Autodesk Inventor part; units mm, degrees
(part 2 of 3)
extrude "Extrusion2" add sketch "Sketch3" against normal blind 0.4 separate body contours L3 L359 L358 L357 L356 L348 L347 L346 L342 L343 L344 L1 L360 L361 L362 L363 L355 L354 L353 L352 L351 L350 | L26 L58 L60 L56 L37 L55 L59 L57 L39 L29 | L67 L70 L63 L171 L170 L162 L163 L72 L164 L161 L71 | L107 L104 L103 L99 L101 L100 L105 L106 L98 | L38 L40 L61 L93 L94 L62 L54 L36 | L73 L78 L168 L82 L166 L167 L165 L83 L74 L81 L80 L79 L77 L76 L75 | L96 L92 A12 A13 L87 | L187 L242 L230 L235 L282 L283 L243 L239 L244 L267 | L270 L271 L272 L274 L276 L277 L278 L275 L273 L268 L269 | L300 L309 L308 L307 L302 L303 L301 L305 L306 | L238 L247 L248 L258 L263 L312 L241 L240 | L249 A39 A42 L262 L264 | L255 L313 L314 L315 L316 L320 L321 L322 L324 L325 L323 L319 L317 L318
sketch "Sketch4" plane through (0, 0, 0.4) normal (0, 0, 1) x (1, 0, 0)
  line L0 (0, 0) -> (63.5, 0)
  line L1 (63.5, 0) -> (63.5, 88.9)
  line L2 (63.5, 88.9) -> (0, 88.9)
  line L3 (0, 88.9) -> (0, 0)
  line L4 (22.2343, 58.9536) -> (21.4951, 58.9536)
  line L5 (22.6153, 59.3346) -> (22.6153, 58.9536)
  line L6 (22.6153, 57.4638) -> (22.6153, 58.9536)
  line L7 (21.4951, 59.3346) -> (22.2343, 59.3346)
  line L8 (21.4951, 52.5322) -> (21.4951, 52.9132)
  line L9 (21.4951, 52.278) -> (21.4951, 58.9536)
  line L10 (21.4951, 52.9132) -> (25.9629, 52.9132)
  line L11 (25.9629, 52.5322) -> (21.4951, 52.5322)
  line L12 (22.6153, 54.7316) -> (22.6153, 57.0828)
  line L13 (22.2343, 58.9536) -> (22.2343, 54.7316)
  circle A0 centre (22.4248, 54.0266) radius 0.3493
  arc A1 (22.2343, 54.7316) -> (22.6153, 54.7316) centre (22.4248, 54.0266) ccw
  line L14 (39.1584, 66.1004) -> (42.0481, 64.4224)
  line L15 (38.6905, 66.1004) -> (39.1584, 66.1004)
  line L16 (38.3095, 62.9084) -> (38.3095, 66.1004)
  line L17 (38.6905, 66.1004) -> (38.6905, 61.5459)
  line L18 (38.3095, 62.9084) -> (37.0962, 62.9084)
  line L19 (37.0962, 62.5274) -> (38.3095, 62.5274)
  line L20 (35.5951, 66.1004) -> (38.3095, 66.1004)
  line L21 (35.2141, 65.0547) -> (35.2141, 66.1004)
  circle A2 centre (38.5, 60.6778) radius 0.508
  circle A3 centre (35.4046, 64.3169) radius 0.3175
  arc A4 (35.2141, 65.0547) -> (35.5951, 65.0547) centre (35.4046, 64.3169) ccw
  line L22 (31.9876, 66.1004) -> (35.2141, 66.1004)
  arc A5 (31.6066, 65.8741) -> (31.9876, 65.8741) centre (31.7971, 65.0383) ccw
  line L23 (35.5951, 66.1004) -> (35.5951, 65.0547)
  line L24 (22.6153, 57.4638) -> (26.9185, 57.4638)
  line L25 (26.9185, 57.0828) -> (22.6153, 57.0828)
  line L26 (26.9185, 57.4638) -> (26.9185, 57.0828)
  circle A6 centre (26.1534, 51.0373) radius 0.4762
  arc A7 (25.9629, 51.8703) -> (26.3439, 51.8703) centre (26.1534, 51.0373) ccw
  line L27 (26.3439, 52.4415) -> (26.3439, 51.8703)
  line L28 (25.9629, 51.8703) -> (25.9629, 52.5322)
  line L29 (26.9185, 55.4481) -> (26.9185, 55.0671)
  line L30 (26.3439, 55.0671) -> (26.3439, 52.8489)
  line L31 (26.9185, 55.0671) -> (26.3439, 55.0671)
  line L32 (25.9629, 52.9132) -> (25.9629, 55.4481)
  line L33 (25.9629, 55.0671) -> (25.9629, 55.4481)
  line L34 (25.9629, 55.4481) -> (26.3439, 55.4481)
  line L35 (25.9629, 55.4481) -> (26.9185, 55.4481)
  line L36 (30.5373, 53.737) -> (30.8468, 54.4929)
  line L37 (29.1789, 54.753) -> (28.0615, 54.753)
  line L38 (29.3943, 53.737) -> (30.5373, 53.737)
  line L39 (26.9185, 54.753) -> (26.9185, 53.737)
  line L40 (29.3943, 53.737) -> (30.8468, 57.9141)
  line L41 (22.2343, 61.6532) -> (25.4283, 64.441)
  line L42 (22.6153, 61.5038) -> (25.4283, 63.959)
  line L43 (25.8093, 61.5568) -> (25.8093, 60.5021)
  line L44 (25.4283, 60.075) -> (25.4283, 60.0896)
  line L45 (25.4283, 60.5021) -> (25.4283, 63.959)
  line L46 (25.8093, 64.9028) -> (25.8093, 61.9378)
  line L47 (25.4283, 64.441) -> (25.4283, 64.9028)
  line L48 (25.4283, 64.9028) -> (22.3363, 64.9028)
  line L49 (21.4951, 59.3346) -> (21.4951, 64.4169)
  line L50 (21.4951, 64.4169) -> (22.3363, 64.9028)
  circle A8 centre (25.6188, 59.7969) radius 0.3493
  line L51 (31.0435, 55.3657) -> (31.9218, 55.3657)
  line L52 (31.4818, 56.4223) -> (31.0435, 55.3657)
  line L53 (31.9218, 55.3657) -> (31.4818, 56.4223)
  line L54 (30.8468, 54.4929) -> (32.1168, 54.4929)
  line L55 (29.1789, 53.737) -> (29.1789, 54.753)
  line L56 (28.0615, 57.9141) -> (28.0615, 54.753)
  line L57 (28.0615, 53.737) -> (26.9185, 53.737)
  line L58 (26.9185, 53.737) -> (26.9185, 57.9141)
  line L59 (26.9185, 53.737) -> (29.1789, 53.737)
  line L60 (26.9185, 57.9141) -> (28.0615, 57.9141)
  line L61 (30.8468, 57.9141) -> (32.1168, 57.9141)
  line L62 (32.4486, 53.737) -> (32.1168, 54.4929)
  line L63 (28.0615, 63.1194) -> (26.9185, 63.1194)
  line L64 (25.8093, 61.9378) -> (26.9185, 61.9378)
  line L65 (26.9185, 61.5568) -> (25.8093, 61.5568)
  line L66 (25.8093, 61.5568) -> (25.8093, 61.6173)
  line L67 (26.9185, 61.9378) -> (26.9185, 61.5568)
  line L68 (22.2343, 59.3346) -> (22.2343, 61.6532)
  line L69 (22.6153, 61.5038) -> (22.6153, 59.3346)
  arc A9 (25.4283, 60.5021) -> (25.8093, 60.5021) centre (25.6188, 59.7969) ccw
  line L70 (26.9185, 63.1194) -> (26.9185, 58.9484)
  line L71 (26.9185, 58.9484) -> (28.0615, 58.9484)
  line L72 (30.9581, 58.9484) -> (29.8151, 58.9484)
  line L73 (32.6087, 58.9484) -> (31.4657, 58.9484)
  line L74 (32.6087, 61.5255) -> (33.8556, 61.5255)
  line L75 (31.4657, 58.9484) -> (33.8556, 58.9484)
  line L76 (33.8556, 58.9484) -> (33.8556, 60.0914)
  line L77 (33.8556, 60.0914) -> (32.6087, 60.0914)
  line L78 (31.4657, 60.0914) -> (31.4657, 58.9484)
  line L79 (32.6087, 60.5095) -> (32.6087, 60.0914)
  line L80 (33.8556, 60.5095) -> (32.6087, 60.5095)
  line L81 (33.8556, 61.5255) -> (33.8556, 60.5095)
  line L82 (31.4657, 60.5095) -> (31.4657, 61.5255)
  line L83 (32.6087, 61.9764) -> (32.6087, 61.5255)
  line L84 (35.0032, 56.9462) -> (35.4388, 56.9462)
  line L85 (35.0032, 54.6929) -> (35.5896, 54.6929)
  line L86 (35.0032, 55.4427) -> (35.5978, 55.4427)
  line L87 (33.911, 53.737) -> (35.876, 53.737)
  line L88 (31.5408, 49.4741) -> (31.5408, 46.3613)
  line L89 (31.9218, 46.3613) -> (31.9218, 48.7095)
  line L90 (31.9218, 46.3613) -> (31.9218, 46.3281)
  line L91 (35.0032, 56.2657) -> (35.0032, 56.9462)
  line L92 (33.911, 57.9141) -> (35.876, 57.9141)
  line L93 (33.5916, 53.737) -> (32.1168, 57.9141)
  line L94 (32.4486, 53.737) -> (33.5916, 53.737)
  line L95 (35.0032, 56.2657) -> (35.4388, 56.2657)
  line L96 (33.911, 53.737) -> (33.911, 57.9141)
  arc A10 (35.4388, 56.2657) -> (35.4388, 56.9462) centre (35.3333, 56.606) ccw
  line L97 (35.0032, 54.6929) -> (35.0032, 55.4427)
  arc A11 (35.5896, 54.6929) -> (35.5978, 55.4427) centre (35.5605, 55.0681) ccw
  arc A12 (36.3387, 56.0044) -> (35.876, 57.9141) centre (35.6477, 56.8479) ccw
  arc A13 (35.876, 53.737) -> (36.3387, 56.0044) centre (35.9369, 54.9055) ccw
  line L98 (37.0962, 62.9084) -> (37.0962, 62.5274)
  line L99 (36.261, 58.9484) -> (35.118, 58.9484)
  line L100 (34.2865, 62.0954) -> (35.118, 62.0954)
  line L101 (35.118, 58.9484) -> (35.118, 62.0954)
  line L102 (35.118, 62.0954) -> (35.2141, 62.0954)
  line L103 (36.261, 62.0954) -> (36.261, 58.9484)
  line L104 (36.261, 62.0954) -> (37.0962, 62.0954)
  line L105 (34.2865, 63.1114) -> (34.2865, 62.0954)
  line L106 (37.0962, 63.1114) -> (34.2865, 63.1114)
  line L107 (37.0962, 62.0954) -> (37.0962, 63.1114)
  line L108 (31.7966, 44.45) -> (43.5019, 51.0525)
  line L109 (42.4624, 51.6596) -> (31.8107, 45.6515)
  line L110 (42.0481, 52.1761) -> (31.9218, 46.3281)
  line L111 (31.9218, 49.1234) -> (37.7054, 52.5185)
  line L112 (31.9218, 48.7095) -> (38.0845, 52.3272)
  line L113 (31.9218, 49.1234) -> (31.9218, 51.0535)
  line L114 (29.0948, 67.2715) -> (29.0948, 67.5351)
  line L115 (29.4758, 67.2715) -> (31.6066, 68.502)
  line L116 (29.0948, 67.5351) -> (31.6066, 68.9857)
  line L117 (31.6066, 65.8741) -> (31.6066, 68.502)
  line L118 (31.6066, 68.9857) -> (31.6066, 70.2564)
  circle A14 centre (29.2853, 63.9396) radius 0.3175
  arc A15 (29.0948, 64.6116) -> (29.4758, 64.6116) centre (29.2853, 63.9396) ccw
  line L119 (29.0948, 64.9028) -> (29.0948, 64.6116)
  line L120 (29.0948, 64.9028) -> (25.8093, 64.9028)
  line L121 (22.9961, 65.2838) -> (29.0948, 65.2838)
  line L122 (29.4758, 64.6116) -> (29.4758, 67.2715)
  line L123 (29.0948, 67.2715) -> (29.0948, 65.2838)
  line L124 (22.9961, 65.2838) -> (31.6066, 70.2564)
  line L125 (31.9876, 66.1004) -> (31.9876, 65.8741)
  line L126 (31.9911, 70.2625) -> (31.9911, 66.4814)
  line L127 (20.9808, 64.9373) -> (31.7409, 71.0066)
  circle A16 centre (31.7971, 65.0383) radius 0.4127
  line L128 (31.75, 72.2052) -> (19.9413, 65.5444)
  line L129 (20.9808, 52.1009) -> (20.9808, 64.9373)
  line L130 (19.9413, 65.5444) -> (19.9413, 51.51)
  circle A17 centre (31.7313, 51.824) radius 0.4127
  line L131 (31.5408, 46.3613) -> (21.4951, 52.278)
  line L132 (19.9413, 51.51) -> (31.7966, 44.45)
  line L133 (31.8107, 45.6515) -> (20.9808, 52.1009)
  line L134 (31.5408, 49.8815) -> (26.3439, 52.8489)
  line L135 (26.3439, 52.4415) -> (31.5408, 49.4741)
  line L136 (31.5408, 51.0535) -> (31.5408, 49.8815)
  arc A18 (31.9218, 51.0535) -> (31.5408, 51.0535) centre (31.7313, 51.824) ccw
  circle A19 centre (41.0606, 62.1232) radius 0.381
  line L137 (40.8701, 59.3346) -> (39.5527, 59.3346)
  line L138 (39.4243, 58.9536) -> (40.8701, 58.9536)
  line L139 (37.7054, 52.5185) -> (37.7054, 53.0908)
  circle A20 centre (37.8959, 53.9267) radius 0.4763
  line L140 (38.7282, 53.737) -> (42.0481, 53.737)
  line L141 (38.0845, 53.0941) -> (38.0845, 52.3272)
  arc A21 (38.7317, 54.1172) -> (37.7054, 53.0908) centre (37.8959, 53.9267) ccw
  arc A22 (38.0845, 53.0941) -> (38.7282, 53.737) centre (37.8959, 53.9267) ccw
  line L142 (42.0481, 53.737) -> (42.0481, 52.1761)
  line L143 (43.5019, 51.0525) -> (43.5019, 65.3384)
  line L144 (42.4624, 64.7418) -> (42.4624, 51.6596)
  line L145 (41.2511, 61.3863) -> (41.2511, 54.1172)
  line L146 (39.4243, 58.9536) -> (38.6183, 59.7969)
  line L147 (39.5527, 59.3346) -> (38.9824, 59.9313)
  arc A23 (41.2511, 61.3863) -> (40.8701, 61.3863) centre (41.0606, 62.1232) ccw
  line L148 (38.3095, 61.5459) -> (38.3095, 62.5274)
  arc A24 (38.9824, 59.9313) -> (38.6905, 61.5459) centre (38.5, 60.6778) ccw
  line L149 (40.8701, 59.3346) -> (40.8701, 61.3863)
  line L150 (42.0481, 64.4224) -> (42.0481, 54.1172)
  line L151 (42.0481, 54.1172) -> (41.2511, 54.1172)
  line L152 (40.8701, 54.1172) -> (40.8701, 58.9536)
  line L153 (40.8701, 54.1172) -> (38.7317, 54.1172)
  arc A25 (38.3095, 61.5459) -> (38.6183, 59.7969) centre (38.5, 60.6778) ccw
  line L154 (43.5019, 65.3384) -> (31.75, 72.2052)
  line L155 (31.7409, 71.0066) -> (42.4624, 64.7418)
  line L156 (38.5023, 66.4814) -> (31.9911, 66.4814)
  line L157 (31.9876, 70.2646) -> (38.5023, 66.4814)
  line L158 (31.9911, 66.4814) -> (31.9911, 70.2625)
  line L159 (31.9911, 70.2625) -> (38.5023, 66.4814)
  line L160 (31.9911, 66.4814) -> (38.5023, 66.4814)
  line L161 (28.0615, 58.9484) -> (28.0615, 61.2883)
  line L162 (29.8151, 63.1194) -> (30.9581, 63.1194)
  line L163 (30.9581, 63.1194) -> (30.9581, 58.9484)
  line L164 (29.8151, 58.9484) -> (28.0615, 61.2883)
  line L165 (33.8556, 61.9764) -> (32.6087, 61.9764)
  line L166 (31.4657, 63.1194) -> (33.8556, 63.1194)
  line L167 (33.8556, 63.1194) -> (33.8556, 61.9764)
  line L168 (31.4657, 58.9484) -> (31.4657, 63.1194)
  line L169 (31.4657, 63.1194) -> (32.6087, 63.1194)
  line L170 (29.8151, 60.7795) -> (29.8151, 63.1194)
  line L171 (28.0615, 63.1194) -> (29.8151, 60.7795)
  line L172 (31.4657, 61.9764) -> (31.4657, 63.1194)
  line L173 (22.6601, 31.2964) -> (22.6651, 29.8066)
  line L174 (22.6665, 29.4256) -> (22.6651, 29.8066)
  line L175 (22.6507, 34.0285) -> (22.6587, 31.6774)
  line L176 (21.5243, 35.8431) -> (25.9921, 35.8584)
  line L177 (25.9908, 36.2394) -> (21.523, 36.2241)
  line L178 (22.2842, 29.8053) -> (21.5449, 29.8027)
  line L179 (21.5462, 29.4217) -> (22.2855, 29.4243)
  circle A26 centre (22.4578, 34.7329) radius 0.3493
  arc A27 (22.6507, 34.0285) -> (22.2697, 34.0272) centre (22.4578, 34.7329) ccw
  line L180 (22.2842, 29.8053) -> (22.2697, 34.0272)
  line L181 (21.523, 36.2241) -> (21.5243, 35.8431)
  line L182 (21.0767, 36.7309) -> (21.12, 24.0813)
  line L183 (19.9676, 23.5047) -> (19.9586, 37.4674)
  line L184 (21.5221, 36.4783) -> (21.5449, 29.8027)
  line L185 (26.9619, 31.6921) -> (22.6587, 31.6774)
  line L186 (22.6601, 31.2964) -> (26.9632, 31.3111)
  line L187 (26.9632, 31.3111) -> (26.9619, 31.6921)
  arc A28 (25.8644, 28.2691) -> (25.4834, 28.2678) centre (25.6715, 28.9736) ccw
  circle A29 centre (25.6715, 28.9736) radius 0.3493
  line L188 (31.8713, 16.6404) -> (19.9676, 23.5047)
  line L189 (21.12, 24.0813) -> (31.8964, 17.907)
  line L190 (23.0676, 23.4777) -> (31.6951, 18.5346)
  line L191 (29.165, 23.8796) -> (29.164, 24.1708)
  line L192 (29.1731, 21.5109) -> (29.1663, 23.4986)
  line L193 (29.1731, 21.5109) -> (29.174, 21.2473)
  line L194 (29.545, 24.1721) -> (29.5541, 21.5122)
  line L195 (29.5541, 21.5122) -> (31.6891, 20.289)
  line L196 (29.174, 21.2473) -> (31.6907, 19.8053)
  line L197 (31.6801, 22.9169) -> (31.6891, 20.289)
  line L198 (31.6907, 19.8053) -> (31.6951, 18.5346)
  line L199 (32.0796, 18.5298) -> (32.0667, 22.3109)
  line L200 (32.0618, 22.6919) -> (32.0611, 22.9182)
  circle A30 centre (31.8677, 23.7534) radius 0.4127
  arc A31 (32.0611, 22.9182) -> (31.6801, 22.9169) centre (31.8677, 23.7534) ccw
  circle A32 centre (41.1212, 26.7001) radius 0.381
  arc A33 (40.9282, 27.4363) -> (41.3092, 27.4376) centre (41.1212, 26.7001) ccw
  line L201 (40.9212, 29.488) -> (40.9282, 27.4363)
  circle A34 centre (38.5556, 28.1368) radius 0.508
  line L202 (40.9212, 29.488) -> (39.6037, 29.4835)
  arc A35 (38.7491, 27.2693) -> (39.0355, 28.8849) centre (38.5556, 28.1368) ccw
  line L203 (39.6037, 29.4835) -> (39.0355, 28.8849)
  line L204 (39.474, 29.8641) -> (40.9199, 29.869)
  line L205 (39.474, 29.8641) -> (38.6709, 29.0181)
  line L206 (42.1166, 24.4043) -> (42.0813, 34.7095)
  line L207 (42.562, 24.1393) -> (42.5183, 36.9086)
  line L208 (43.6866, 37.5937) -> (43.6957, 23.5059)
  line L209 (41.3092, 27.4376) -> (41.2843, 34.7068)
  line L210 (40.9033, 34.7055) -> (40.9199, 29.869)
  line L211 (38.7601, 35.0783) -> (42.08, 35.0897)
  line L212 (40.9033, 34.7055) -> (38.7649, 34.6981)
  line L213 (26.9772, 27.2181) -> (25.868, 27.2143)
  line L214 (25.8693, 26.8333) -> (26.9785, 26.8371)
  line L215 (25.868, 27.2143) -> (25.8644, 28.2691)
  line L216 (25.868, 27.2143) -> (25.8682, 27.1538)
  line L217 (22.6739, 27.2564) -> (22.6665, 29.4256)
  line L218 (22.2855, 29.4243) -> (22.2934, 27.1057)
  line L219 (25.4834, 28.2678) -> (25.4952, 24.8108)
  line L220 (22.6739, 27.2564) -> (25.4952, 24.8108)
  line L221 (21.5462, 29.4217) -> (21.5636, 24.3395)
  line L222 (25.8795, 23.8684) -> (25.8693, 26.8333)
  line L223 (25.4985, 23.8671) -> (22.4066, 23.8565)
  line L224 (21.5636, 24.3395) -> (22.4066, 23.8565)
  line L225 (22.2934, 27.1057) -> (25.4969, 24.3288)
  line L226 (25.9921, 35.8584) -> (26.0007, 33.3235)
  line L227 (26.3804, 33.7058) -> (26.3728, 35.924)
  line L228 (25.9885, 36.9013) -> (25.9908, 36.2394)
  line L229 (26.3714, 36.3314) -> (26.3695, 36.9026)
  line L230 (26.9563, 33.3268) -> (26.955, 33.7078)
  line L231 (26.955, 33.7078) -> (26.3804, 33.7058)
  line L232 (25.9994, 33.7045) -> (26.0007, 33.3235)
  line L233 (26.0007, 33.3235) -> (26.3817, 33.3248)
  line L234 (26.0007, 33.3235) -> (26.9563, 33.3268)
  line L235 (26.954, 34.0219) -> (26.9505, 35.0379)
  line L236 (25.4819, 28.6948) -> (25.482, 28.6802)
  line L237 (25.4969, 24.3288) -> (25.4985, 23.8671)
  line L238 (30.5693, 35.0503) -> (30.8814, 34.2954)
  line L239 (29.2143, 34.0297) -> (28.097, 34.0258)
  line L240 (29.4263, 35.0464) -> (30.5693, 35.0503)
  line L241 (29.4263, 35.0464) -> (30.8931, 30.8743)
  line L242 (26.9505, 35.0379) -> (26.9648, 30.8608)
  line L243 (29.2108, 35.0457) -> (29.2143, 34.0297)
  line L244 (28.1078, 30.8647) -> (28.097, 34.0258)
  circle A36 centre (31.7568, 36.9673) radius 0.4127
  line L245 (31.9366, 40.0825) -> (38.1116, 36.4859)
  line L246 (31.938, 39.6686) -> (37.7332, 36.2932)
  line L247 (30.8814, 34.2954) -> (32.1514, 34.2998)
  line L248 (32.4805, 35.0569) -> (32.1514, 34.2998)
  line L249 (33.9429, 35.0619) -> (35.9079, 35.0686)
  line L250 (31.081, 33.4233) -> (31.9594, 33.4263)
  line L251 (31.523, 32.3682) -> (31.081, 33.4233)
  line L252 (31.9594, 33.4263) -> (31.523, 32.3682)
  line L253 (35.0384, 34.1097) -> (35.6249, 34.1117)
  line L254 (35.041, 33.3599) -> (35.6356, 33.3619)
  circle A37 centre (37.9285, 34.8858) radius 0.4763
  arc A38 (37.7351, 35.7209) -> (38.7649, 34.6981) centre (37.9285, 34.8858) ccw
  arc A39 (36.3784, 32.8027) -> (35.9079, 35.0686) centre (35.9728, 33.9003) ccw
  line L255 (33.9054, 29.8503) -> (33.9093, 28.7073)
  line L256 (31.938, 39.6686) -> (31.9446, 37.7385)
  line L257 (35.0461, 31.8563) -> (35.4817, 31.8578)
  line L258 (32.4805, 35.0569) -> (33.6235, 35.0608)
  line L259 (35.0438, 32.5368) -> (35.4794, 32.5383)
  line L260 (35.0384, 34.1097) -> (35.041, 33.3599)
  arc A40 (35.6356, 33.3619) -> (35.6249, 34.1117) centre (35.597, 33.7363) ccw
  line L261 (35.0438, 32.5368) -> (35.0461, 31.8563)
  arc A41 (35.4817, 31.8578) -> (35.4794, 32.5383) centre (35.375, 32.1977) ccw
  arc A42 (35.9222, 30.8915) -> (36.3784, 32.8027) centre (35.6902, 31.9569) ccw
  line L262 (33.9572, 30.8847) -> (35.9222, 30.8915)
  line L263 (33.6235, 35.0608) -> (32.1631, 30.8786)
  line L264 (33.9429, 35.0619) -> (33.9572, 30.8847)
  line L265 (42.0813, 34.7095) -> (41.2843, 34.7068)
  line L266 (42.08, 35.0897) -> (42.0747, 36.6505)
  line L267 (26.9648, 30.8608) -> (28.1078, 30.8647)
  line L268 (28.1256, 25.6594) -> (26.9826, 25.6555)
  line L269 (26.9785, 26.8371) -> (26.9772, 27.2181)
  line L270 (26.9826, 25.6555) -> (26.9683, 29.8265)
  line L271 (26.9683, 29.8265) -> (28.1113, 29.8304)
  line L272 (28.1113, 29.8304) -> (28.1193, 27.4905)
  line L273 (28.1256, 25.6594) -> (29.8712, 28.0053)
  line L274 (29.8649, 29.8364) -> (28.1193, 27.4905)
  line L275 (29.8712, 28.0053) -> (29.8792, 25.6654)
  line L276 (31.0079, 29.8403) -> (29.8649, 29.8364)
  line L277 (31.0222, 25.6693) -> (31.0079, 29.8403)
  circle A43 centre (29.3522, 24.8434) radius 0.3175
  line L278 (29.8792, 25.6654) -> (31.0222, 25.6693)
  arc A44 (29.545, 24.1721) -> (29.164, 24.1708) centre (29.3522, 24.8434) ccw
  line L279 (38.3728, 25.9055) -> (38.3837, 22.7135)
  line L280 (38.7647, 22.7148) -> (38.7491, 27.2693)
  line L281 (38.3681, 27.268) -> (38.3715, 26.2865)
  circle A45 centre (26.1761, 37.735) radius 0.4762
  arc A46 (26.3695, 36.9026) -> (25.9885, 36.9013) centre (26.1761, 37.735) ccw
  line L282 (28.0935, 35.0418) -> (26.9505, 35.0379)
  line L283 (26.9505, 35.0379) -> (29.2108, 35.0457)
  line L284 (31.5582, 39.3166) -> (31.5476, 42.4293)
  line L285 (31.5596, 38.9092) -> (26.3728, 35.924)
  line L286 (26.3714, 36.3314) -> (31.5582, 39.3166)
  line L287 (31.5476, 42.4293) -> (21.5221, 36.4783)
  line L288 (31.7603, 43.0725) -> (21.0767, 36.7309)
  line L289 (19.9586, 37.4674) -> (31.7966, 44.45)
  line L290 (31.9286, 42.4307) -> (31.9366, 40.0825)
  line L291 (31.9286, 42.4307) -> (31.9285, 42.4639)
  line L292 (31.7966, 44.45) -> (43.6866, 37.5937)
  line L293 (42.5183, 36.9086) -> (31.7603, 43.0725)
  line L294 (42.0747, 36.6505) -> (31.9285, 42.4639)
  line L295 (31.5636, 37.7372) -> (31.5596, 38.9092)
  arc A47 (31.5636, 37.7372) -> (31.9446, 37.7385) centre (31.7568, 36.9673) ccw
  line L296 (38.1142, 35.719) -> (38.1116, 36.4859)
  arc A48 (38.7601, 35.0783) -> (38.1142, 35.719) centre (37.9285, 34.8858) ccw
  line L297 (37.7332, 36.2932) -> (37.7351, 35.7209)
  line L298 (38.3728, 25.9055) -> (37.1595, 25.9014)
  line L299 (37.1582, 26.2824) -> (38.3715, 26.2865)
  line L300 (37.1595, 25.9014) -> (37.1582, 26.2824)
  line L301 (36.3108, 29.8585) -> (35.1678, 29.8546)
  line L302 (34.347, 26.7047) -> (35.1786, 26.7075)
  line L303 (35.1678, 29.8546) -> (35.1786, 26.7075)
  line L304 (35.1786, 26.7075) -> (35.2746, 26.7079)
  line L305 (36.3215, 26.7115) -> (36.3108, 29.8585)
  line L306 (36.3215, 26.7115) -> (37.1567, 26.7143)
  line L307 (34.3505, 25.6887) -> (34.347, 26.7047)
  line L308 (37.1602, 25.6983) -> (34.3505, 25.6887)
  line L309 (37.1567, 26.7143) -> (37.1602, 25.6983)
  arc A49 (38.6709, 29.0181) -> (38.3681, 27.268) centre (38.5556, 28.1368) ccw
  line L310 (29.165, 23.8796) -> (25.8795, 23.8684)
  line L311 (23.0676, 23.4777) -> (29.1663, 23.4986)
  line L312 (30.8931, 30.8743) -> (32.1631, 30.8786)
  line L313 (33.9093, 28.7073) -> (32.6624, 28.703)
  line L314 (32.6638, 28.2849) -> (32.6624, 28.703)
  line L315 (33.9107, 28.2892) -> (32.6638, 28.2849)
  line L316 (33.9142, 27.2732) -> (33.9107, 28.2892)
  line L317 (32.6585, 29.846) -> (31.5155, 29.8421)
  line L318 (31.5155, 29.8421) -> (33.9054, 29.8503)
  line L319 (31.5194, 28.6991) -> (31.5155, 29.8421)
  line L320 (32.6673, 27.2689) -> (33.9142, 27.2732)
  line L321 (32.6688, 26.818) -> (32.6673, 27.2689)
  line L322 (33.9158, 26.8222) -> (32.6688, 26.818)
  line L323 (31.5155, 29.8421) -> (31.5298, 25.6711)
  line L324 (33.9197, 25.6792) -> (33.9158, 26.8222)
  line L325 (31.5298, 25.6711) -> (33.9197, 25.6792)
  line L326 (31.5298, 25.6711) -> (32.6728, 25.675)
  line L327 (31.5258, 26.8141) -> (31.5298, 25.6711)
  line L328 (31.5208, 28.281) -> (31.5243, 27.265)
  line L329 (39.2326, 22.7164) -> (42.1166, 24.4043)
  line L330 (38.7647, 22.7148) -> (39.2326, 22.7164)
  line L331 (35.6693, 22.7042) -> (38.3837, 22.7135)
  line L332 (35.2848, 23.7486) -> (35.2883, 22.7029)
  circle A50 centre (35.4727, 24.4871) radius 0.3175
  arc A51 (35.6658, 23.7499) -> (35.2848, 23.7486) centre (35.4727, 24.4871) ccw
  line L333 (32.0618, 22.6919) -> (35.2883, 22.7029)
  line L334 (35.6693, 22.7042) -> (35.6658, 23.7499)
  line L335 (38.5779, 22.3332) -> (32.0667, 22.3109)
  line L336 (32.0667, 22.3109) -> (38.5779, 22.3332)
  line L337 (31.8964, 17.907) -> (42.562, 24.1393)
  line L338 (43.6957, 23.5059) -> (31.8713, 16.6404)
  line L339 (32.0796, 18.5298) -> (38.5779, 22.3332)
  line L340 (32.0761, 18.5277) -> (38.5779, 22.3332)
  line L341 (32.0667, 22.3109) -> (32.0796, 18.5298)
  line L342 (31.75, 80.4139) -> (44.6823, 72.8573)
  line L343 (44.6823, 72.8573) -> (54.0323, 76.3351)
  line L344 (54.0323, 76.3351) -> (63.5, 70.8029)
  line L345 (31.75, 72.2052) -> (31.75, 88.9) construction
  line L346 (31.75, 80.4139) -> (18.8177, 72.8573)
  line L347 (18.8177, 72.8573) -> (9.4677, 76.3351)
  line L348 (9.4677, 76.3351) -> (0, 70.8029)
  line L349 (29.1432, 44.45) -> (63.5, 44.45) construction
  line L350 (9.4677, 12.5649) -> (0, 18.0971)
  line L351 (18.8177, 16.0427) -> (9.4677, 12.5649)
  line L352 (31.75, 8.4861) -> (18.8177, 16.0427)
  line L353 (31.75, 8.4861) -> (44.6823, 16.0427)
  line L354 (44.6823, 16.0427) -> (54.0323, 12.5649)
  line L355 (54.0323, 12.5649) -> (63.5, 18.0971)
  line L356 (0, 51.1737) -> (17.8526, 51.1737)
  line L357 (17.8526, 51.1737) -> (29.1432, 44.45)
  line L358 (17.8526, 37.7263) -> (29.1432, 44.45)
  line L359 (0, 37.7263) -> (17.8526, 37.7263)
  line L360 (63.5, 51.1737) -> (45.6474, 51.1737)
  line L361 (45.6474, 51.1737) -> (34.3568, 44.45)
  line L362 (45.6474, 37.7263) -> (34.3568, 44.45)
  line L363 (63.5, 37.7263) -> (45.6474, 37.7263)
  point P0 (0, 0)
  point P1 (31.7785, 58.3278)
  point P2 (31.8262, 30.4638)
  point P3 (-41.3099, 18.32)
  point P4 (-51.7367, 24.4909)
  point P5 (-46.8879, 27.4068)
  point P6 (-46.3133, 27.4068)
  point P7 (-46.3133, 29.0414)
  point P8 (-41.2407, 42.2212)
  point P9 (-46.3133, 29.4224)
  point P10 (-45.1703, 25.6956)
  point P11 (-46.3133, 26.7116)
  point P12 (-46.3133, 27.0258)
  point P13 (-36.1356, 34.4861)
  point P14 (-36.1356, 34.8671)
  point P15 (-46.3133, 33.8965)
  point P16 (-46.3133, 33.5155)
  point P17 (-40.6231, 30.9071)
  point P18 (-41.7661, 32.0501)
  point P19 (-41.7661, 32.4682)
  point P20 (-41.3032, 14.3893)
  point P21 (-51.7088, 8.1828)
  point P22 (-46.2698, 3.6508)
  point P23 (-46.2754, 5.2854)
  point P24 (-46.85, 5.2835)
  point P25 (-46.2545, -0.8232)
  point P26 (-46.2532, -1.2042)
  point P27 (-36.0723, -2.1399)
  point P28 (-36.0736, -1.7589)
  point P29 (-46.2767, 5.6664)
  point P30 (-46.2778, 5.9806)
  point P31 (-45.1383, 7.0005)
  point P32 (-46.2685, 3.2698)
  point P33 (-41.7124, 0.6578)
  point P34 (-40.5733, 1.8047)
  point P35 (-9.7318, -9.9442)
  point P36 (-73.2318, -9.9442)
  point P37 (-73.2318, 42.7616)
  dimension "d21" = 63.5
  dimension "d22" = 88.9
  constraints: 728 end point, 89 parallel, 64 point on circle, 50 centre point, 37 horizontal, 22 point on line, 21 perpendicular, 20 coincident, 17 symmetric about line, 5 vertical, 4 collinear, 2 midpoint, 11 other
  measures "d21" distance of L2.end L1.end
  measures "d22" distance of L1.end L0.end
extrude "Extrusion3" add sketch "Sketch4" against normal blind 0.4 separate body contours L3 L356 L357 L358 L359 | L363 L362 L361 L360 L1
sketch "Sketch5" plane through (0, 0, 0) normal (0, 0, -1) x (-1, 0, 0)
  line L0 (-29.8712, 28.0053) -> (-28.1256, 25.6594) projected
  line L1 (-28.1256, 25.6594) -> (-26.9826, 25.6555) projected
  line L2 (-26.9826, 25.6555) -> (-26.9683, 29.8265) projected
  line L3 (-26.9683, 29.8265) -> (-28.1113, 29.8304) projected
  line L4 (-28.1113, 29.8304) -> (-28.1193, 27.4905) projected
  line L5 (-28.1193, 27.4905) -> (-29.8649, 29.8364) projected
  line L6 (-29.8649, 29.8364) -> (-31.0079, 29.8403) projected
  line L7 (-31.0079, 29.8403) -> (-31.0222, 25.6693) projected
  line L8 (-31.0222, 25.6693) -> (-29.8792, 25.6654) projected
  line L9 (-29.8792, 25.6654) -> (-29.8712, 28.0053) projected
  line L10 (-28.097, 34.0258) -> (-28.1078, 30.8647) projected
  line L11 (-28.1078, 30.8647) -> (-26.9648, 30.8608) projected
  line L12 (-26.9648, 30.8608) -> (-26.9505, 35.0379) projected
  line L13 (-26.9505, 35.0379) -> (-29.2108, 35.0457) projected
  line L14 (-29.2108, 35.0457) -> (-29.2143, 34.0297) projected
  line L15 (-29.2143, 34.0297) -> (-28.097, 34.0258) projected
  line L16 (-32.1631, 30.8786) -> (-30.8931, 30.8743) projected
  line L17 (-30.8931, 30.8743) -> (-29.4263, 35.0464) projected
  line L18 (-29.4263, 35.0464) -> (-30.5693, 35.0503) projected
  line L19 (-30.5693, 35.0503) -> (-30.8814, 34.2954) projected
  line L20 (-30.8814, 34.2954) -> (-32.1514, 34.2998) projected
  line L21 (-32.1514, 34.2998) -> (-32.4805, 35.0569) projected
  line L22 (-32.4805, 35.0569) -> (-33.6235, 35.0608) projected
  line L23 (-33.6235, 35.0608) -> (-32.1631, 30.8786) projected
  line L24 (-31.9594, 33.4263) -> (-31.081, 33.4233) projected
  line L25 (-31.081, 33.4233) -> (-31.523, 32.3682) projected
  line L26 (-31.523, 32.3682) -> (-31.9594, 33.4263) projected
  arc A0 (-36.3784, 32.8027) -> (-35.9222, 30.8915) centre (-35.6902, 31.9569) ccw projected
  line L27 (-35.9222, 30.8915) -> (-33.9572, 30.8847) projected
  line L28 (-33.9572, 30.8847) -> (-33.9429, 35.0619) projected
  line L29 (-33.9429, 35.0619) -> (-35.9079, 35.0686) projected
  arc A1 (-35.9079, 35.0686) -> (-36.3784, 32.8027) centre (-35.9728, 33.9003) ccw projected
  line L30 (-35.4794, 32.5383) -> (-35.0438, 32.5368) projected
  line L31 (-35.0438, 32.5368) -> (-35.0461, 31.8563) projected
  line L32 (-35.0461, 31.8563) -> (-35.4817, 31.8578) projected
  arc A2 (-35.4794, 32.5383) -> (-35.4817, 31.8578) centre (-35.375, 32.1977) ccw projected
  line L33 (-35.0384, 34.1097) -> (-35.041, 33.3599) projected
  line L34 (-35.041, 33.3599) -> (-35.6356, 33.3619) projected
  arc A3 (-35.6249, 34.1117) -> (-35.6356, 33.3619) centre (-35.597, 33.7363) ccw projected
  line L35 (-35.6249, 34.1117) -> (-35.0384, 34.1097) projected
  line L36 (-31.5155, 29.8421) -> (-33.9054, 29.8503) projected
  line L37 (-33.9054, 29.8503) -> (-33.9093, 28.7073) projected
  line L38 (-33.9093, 28.7073) -> (-32.6624, 28.703) projected
  line L39 (-32.6624, 28.703) -> (-32.6638, 28.2849) projected
  line L40 (-32.6638, 28.2849) -> (-33.9107, 28.2892) projected
  line L41 (-33.9107, 28.2892) -> (-33.9142, 27.2732) projected
  line L42 (-33.9142, 27.2732) -> (-32.6673, 27.2689) projected
  line L43 (-32.6673, 27.2689) -> (-32.6688, 26.818) projected
  line L44 (-32.6688, 26.818) -> (-33.9158, 26.8222) projected
  line L45 (-33.9158, 26.8222) -> (-33.9197, 25.6792) projected
  line L46 (-33.9197, 25.6792) -> (-31.5298, 25.6711) projected
  line L47 (-31.5298, 25.6711) -> (-31.5155, 29.8421) projected
  line L48 (-36.3108, 29.8585) -> (-36.3215, 26.7115) projected
  line L49 (-36.3215, 26.7115) -> (-37.1567, 26.7143) projected
  line L50 (-37.1567, 26.7143) -> (-37.1602, 25.6983) projected
  line L51 (-37.1602, 25.6983) -> (-34.3505, 25.6887) projected
  line L52 (-34.3505, 25.6887) -> (-34.347, 26.7047) projected
  line L53 (-34.347, 26.7047) -> (-35.1786, 26.7075) projected
  line L54 (-35.1786, 26.7075) -> (-35.1678, 29.8546) projected
  line L55 (-35.1678, 29.8546) -> (-36.3108, 29.8585) projected
  line L56 (-26.9185, 58.9484) -> (-26.9185, 63.1194) projected
  line L57 (-26.9185, 63.1194) -> (-28.0615, 63.1194) projected
  line L58 (-28.0615, 63.1194) -> (-29.8151, 60.7795) projected
  line L59 (-29.8151, 60.7795) -> (-29.8151, 63.1194) projected
  line L60 (-29.8151, 63.1194) -> (-30.9581, 63.1194) projected
  line L61 (-30.9581, 63.1194) -> (-30.9581, 58.9484) projected
  line L62 (-30.9581, 58.9484) -> (-29.8151, 58.9484) projected
  line L63 (-29.8151, 58.9484) -> (-28.0615, 61.2883) projected
  line L64 (-28.0615, 61.2883) -> (-28.0615, 58.9484) projected
  line L65 (-28.0615, 58.9484) -> (-26.9185, 58.9484) projected
  line L66 (-32.6087, 60.0914) -> (-33.8556, 60.0914) projected
  line L67 (-33.8556, 60.0914) -> (-33.8556, 58.9484) projected
  line L68 (-33.8556, 58.9484) -> (-31.4657, 58.9484) projected
  line L69 (-31.4657, 58.9484) -> (-31.4657, 63.1194) projected
  line L70 (-31.4657, 63.1194) -> (-33.8556, 63.1194) projected
  line L71 (-33.8556, 63.1194) -> (-33.8556, 61.9764) projected
  line L72 (-33.8556, 61.9764) -> (-32.6087, 61.9764) projected
  line L73 (-32.6087, 61.9764) -> (-32.6087, 61.5255) projected
  line L74 (-32.6087, 61.5255) -> (-33.8556, 61.5255) projected
  line L75 (-33.8556, 61.5255) -> (-33.8556, 60.5095) projected
  line L76 (-33.8556, 60.5095) -> (-32.6087, 60.5095) projected
  line L77 (-32.6087, 60.5095) -> (-32.6087, 60.0914) projected
  line L78 (-37.0962, 63.1114) -> (-37.0962, 62.0954) projected
  line L79 (-37.0962, 62.0954) -> (-36.261, 62.0954) projected
  line L80 (-36.261, 62.0954) -> (-36.261, 58.9484) projected
  line L81 (-36.261, 58.9484) -> (-35.118, 58.9484) projected
  line L82 (-35.118, 58.9484) -> (-35.118, 62.0954) projected
  line L83 (-35.118, 62.0954) -> (-34.2865, 62.0954) projected
  line L84 (-34.2865, 62.0954) -> (-34.2865, 63.1114) projected
  line L85 (-34.2865, 63.1114) -> (-37.0962, 63.1114) projected
  line L86 (-26.9185, 53.737) -> (-26.9185, 57.9141) projected
  line L87 (-26.9185, 57.9141) -> (-28.0615, 57.9141) projected
  line L88 (-28.0615, 57.9141) -> (-28.0615, 54.753) projected
  line L89 (-28.0615, 54.753) -> (-29.1789, 54.753) projected
  line L90 (-29.1789, 54.753) -> (-29.1789, 53.737) projected
  line L91 (-29.1789, 53.737) -> (-26.9185, 53.737) projected
  line L92 (-30.8468, 54.4929) -> (-30.5373, 53.737) projected
  line L93 (-30.5373, 53.737) -> (-29.3943, 53.737) projected
  line L94 (-29.3943, 53.737) -> (-30.8468, 57.9141) projected
  line L95 (-30.8468, 57.9141) -> (-32.1168, 57.9141) projected
  line L96 (-32.1168, 57.9141) -> (-33.5916, 53.737) projected
  line L97 (-33.5916, 53.737) -> (-32.4486, 53.737) projected
  line L98 (-32.4486, 53.737) -> (-32.1168, 54.4929) projected
  line L99 (-32.1168, 54.4929) -> (-30.8468, 54.4929) projected
  line L100 (-31.4818, 56.4223) -> (-31.0435, 55.3657) projected
  line L101 (-31.0435, 55.3657) -> (-31.9218, 55.3657) projected
  line L102 (-31.9218, 55.3657) -> (-31.4818, 56.4223) projected
  line L103 (-35.876, 53.737) -> (-33.911, 53.737) projected
  line L104 (-33.911, 53.737) -> (-33.911, 57.9141) projected
  line L105 (-33.911, 57.9141) -> (-35.876, 57.9141) projected
  arc A4 (-35.876, 57.9141) -> (-36.3387, 56.0044) centre (-35.6477, 56.8479) ccw projected
  arc A5 (-36.3387, 56.0044) -> (-35.876, 53.737) centre (-35.9369, 54.9055) ccw projected
  line L106 (-35.5978, 55.4427) -> (-35.0032, 55.4427) projected
  line L107 (-35.0032, 55.4427) -> (-35.0032, 54.6929) projected
  line L108 (-35.0032, 54.6929) -> (-35.5896, 54.6929) projected
  arc A6 (-35.5978, 55.4427) -> (-35.5896, 54.6929) centre (-35.5605, 55.0681) ccw projected
  line L109 (-35.0032, 56.9462) -> (-35.0032, 56.2657) projected
  line L110 (-35.0032, 56.2657) -> (-35.4388, 56.2657) projected
  arc A7 (-35.4388, 56.9462) -> (-35.4388, 56.2657) centre (-35.3333, 56.606) ccw projected
  line L111 (-35.4388, 56.9462) -> (-35.0032, 56.9462) projected
  point P0 (0, 0)
extrude "Extrusion4" add sketch "Sketch5" along normal blind 0.4 bodies 2
sketch "Sketch6" plane through (0, 0, 0.4) normal (0, 0, 1) x (1, 0, 0)
  line L0 (0, 0) -> (63.5, 0)
  line L1 (63.5, 0) -> (63.5, 88.9)
  line L2 (63.5, 88.9) -> (0, 88.9)
  line L3 (0, 88.9) -> (0, 0)
  line L4 (22.2343, 58.9536) -> (21.4951, 58.9536)
  line L5 (22.6153, 59.3346) -> (22.6153, 58.9536)
  line L6 (22.6153, 57.4638) -> (22.6153, 58.9536)
  line L7 (21.4951, 59.3346) -> (22.2343, 59.3346)
  line L8 (21.4951, 52.5322) -> (21.4951, 52.9132)
  line L9 (21.4951, 52.278) -> (21.4951, 58.9536)
  line L10 (21.4951, 52.9132) -> (25.9629, 52.9132)
  line L11 (25.9629, 52.5322) -> (21.4951, 52.5322)
  line L12 (22.6153, 54.7316) -> (22.6153, 57.0828)
  line L13 (22.2343, 58.9536) -> (22.2343, 54.7316)
  circle A0 centre (22.4248, 54.0266) radius 0.3493
  arc A1 (22.2343, 54.7316) -> (22.6153, 54.7316) centre (22.4248, 54.0266) ccw
  line L14 (39.1584, 66.1004) -> (42.0481, 64.4224)
  line L15 (38.6905, 66.1004) -> (39.1584, 66.1004)
  line L16 (38.3095, 62.9084) -> (38.3095, 66.1004)
  line L17 (38.6905, 66.1004) -> (38.6905, 61.5459)
  line L18 (38.3095, 62.9084) -> (37.0962, 62.9084)
  line L19 (37.0962, 62.5274) -> (38.3095, 62.5274)
  line L20 (35.5951, 66.1004) -> (38.3095, 66.1004)
  line L21 (35.2141, 65.0547) -> (35.2141, 66.1004)
  circle A2 centre (38.5, 60.6778) radius 0.508
  circle A3 centre (35.4046, 64.3169) radius 0.3175
  arc A4 (35.2141, 65.0547) -> (35.5951, 65.0547) centre (35.4046, 64.3169) ccw
  line L22 (31.9876, 66.1004) -> (35.2141, 66.1004)
  arc A5 (31.6066, 65.8741) -> (31.9876, 65.8741) centre (31.7971, 65.0383) ccw
  line L23 (35.5951, 66.1004) -> (35.5951, 65.0547)
  line L24 (22.6153, 57.4638) -> (26.9185, 57.4638)
  line L25 (26.9185, 57.0828) -> (22.6153, 57.0828)
  line L26 (26.9185, 57.4638) -> (26.9185, 57.0828)
  circle A6 centre (26.1534, 51.0373) radius 0.4762
  arc A7 (25.9629, 51.8703) -> (26.3439, 51.8703) centre (26.1534, 51.0373) ccw
  line L27 (26.3439, 52.4415) -> (26.3439, 51.8703)
  line L28 (25.9629, 51.8703) -> (25.9629, 52.5322)
  line L29 (26.9185, 55.4481) -> (26.9185, 55.0671)
  line L30 (26.3439, 55.0671) -> (26.3439, 52.8489)
  line L31 (26.9185, 55.0671) -> (26.3439, 55.0671)
  line L32 (25.9629, 52.9132) -> (25.9629, 55.4481)
  line L33 (25.9629, 55.0671) -> (25.9629, 55.4481)
  line L34 (25.9629, 55.4481) -> (26.3439, 55.4481)
  line L35 (25.9629, 55.4481) -> (26.9185, 55.4481)
  line L36 (30.5373, 53.737) -> (30.8468, 54.4929)
  line L37 (29.1789, 54.753) -> (28.0615, 54.753)
  line L38 (29.3943, 53.737) -> (30.5373, 53.737)
  line L39 (26.9185, 54.753) -> (26.9185, 53.737)
  line L40 (29.3943, 53.737) -> (30.8468, 57.9141)
  line L41 (22.2343, 61.6532) -> (25.4283, 64.441)
  line L42 (22.6153, 61.5038) -> (25.4283, 63.959)
  line L43 (25.8093, 61.5568) -> (25.8093, 60.5021)
  line L44 (25.4283, 60.075) -> (25.4283, 60.0896)
  line L45 (25.4283, 60.5021) -> (25.4283, 63.959)
  line L46 (25.8093, 64.9028) -> (25.8093, 61.9378)
  line L47 (25.4283, 64.441) -> (25.4283, 64.9028)
  line L48 (25.4283, 64.9028) -> (22.3363, 64.9028)
  line L49 (21.4951, 59.3346) -> (21.4951, 64.4169)
  line L50 (21.4951, 64.4169) -> (22.3363, 64.9028)
  circle A8 centre (25.6188, 59.7969) radius 0.3493
  line L51 (31.0435, 55.3657) -> (31.9218, 55.3657)
  line L52 (31.4818, 56.4223) -> (31.0435, 55.3657)
  line L53 (31.9218, 55.3657) -> (31.4818, 56.4223)
  line L54 (30.8468, 54.4929) -> (32.1168, 54.4929)
  line L55 (29.1789, 53.737) -> (29.1789, 54.753)
  line L56 (28.0615, 57.9141) -> (28.0615, 54.753)
  line L57 (28.0615, 53.737) -> (26.9185, 53.737)
  line L58 (26.9185, 53.737) -> (26.9185, 57.9141)
  line L59 (26.9185, 53.737) -> (29.1789, 53.737)
  line L60 (26.9185, 57.9141) -> (28.0615, 57.9141)
  line L61 (30.8468, 57.9141) -> (32.1168, 57.9141)
  line L62 (32.4486, 53.737) -> (32.1168, 54.4929)
  line L63 (28.0615, 63.1194) -> (26.9185, 63.1194)
  line L64 (25.8093, 61.9378) -> (26.9185, 61.9378)
  line L65 (26.9185, 61.5568) -> (25.8093, 61.5568)
  line L66 (25.8093, 61.5568) -> (25.8093, 61.6173)
  line L67 (26.9185, 61.9378) -> (26.9185, 61.5568)
  line L68 (22.2343, 59.3346) -> (22.2343, 61.6532)
  line L69 (22.6153, 61.5038) -> (22.6153, 59.3346)
  arc A9 (25.4283, 60.5021) -> (25.8093, 60.5021) centre (25.6188, 59.7969) ccw
  line L70 (26.9185, 63.1194) -> (26.9185, 58.9484)
  line L71 (26.9185, 58.9484) -> (28.0615, 58.9484)
  line L72 (30.9581, 58.9484) -> (29.8151, 58.9484)
  line L73 (32.6087, 58.9484) -> (31.4657, 58.9484)
  line L74 (32.6087, 61.5255) -> (33.8556, 61.5255)
  line L75 (31.4657, 58.9484) -> (33.8556, 58.9484)
  line L76 (33.8556, 58.9484) -> (33.8556, 60.0914)
  line L77 (33.8556, 60.0914) -> (32.6087, 60.0914)
  line L78 (31.4657, 60.0914) -> (31.4657, 58.9484)
  line L79 (32.6087, 60.5095) -> (32.6087, 60.0914)
  line L80 (33.8556, 60.5095) -> (32.6087, 60.5095)
  line L81 (33.8556, 61.5255) -> (33.8556, 60.5095)
  line L82 (31.4657, 60.5095) -> (31.4657, 61.5255)
  line L83 (32.6087, 61.9764) -> (32.6087, 61.5255)
  line L84 (35.0032, 56.9462) -> (35.4388, 56.9462)
  line L85 (35.0032, 54.6929) -> (35.5896, 54.6929)
  line L86 (35.0032, 55.4427) -> (35.5978, 55.4427)
  line L87 (33.911, 53.737) -> (35.876, 53.737)
  line L88 (31.5408, 49.4741) -> (31.5408, 46.3613)
  line L89 (31.9218, 46.3613) -> (31.9218, 48.7095)
  line L90 (31.9218, 46.3613) -> (31.9218, 46.3281)
  line L91 (35.0032, 56.2657) -> (35.0032, 56.9462)
  line L92 (33.911, 57.9141) -> (35.876, 57.9141)
  line L93 (33.5916, 53.737) -> (32.1168, 57.9141)
  line L94 (32.4486, 53.737) -> (33.5916, 53.737)
  line L95 (35.0032, 56.2657) -> (35.4388, 56.2657)
  line L96 (33.911, 53.737) -> (33.911, 57.9141)
  arc A10 (35.4388, 56.2657) -> (35.4388, 56.9462) centre (35.3333, 56.606) ccw
  line L97 (35.0032, 54.6929) -> (35.0032, 55.4427)
  arc A11 (35.5896, 54.6929) -> (35.5978, 55.4427) centre (35.5605, 55.0681) ccw
  arc A12 (36.3387, 56.0044) -> (35.876, 57.9141) centre (35.6477, 56.8479) ccw
  arc A13 (35.876, 53.737) -> (36.3387, 56.0044) centre (35.9369, 54.9055) ccw
  line L98 (37.0962, 62.9084) -> (37.0962, 62.5274)
  line L99 (36.261, 58.9484) -> (35.118, 58.9484)
  line L100 (34.2865, 62.0954) -> (35.118, 62.0954)
  line L101 (35.118, 58.9484) -> (35.118, 62.0954)
  line L102 (35.118, 62.0954) -> (35.2141, 62.0954)
  line L103 (36.261, 62.0954) -> (36.261, 58.9484)
  line L104 (36.261, 62.0954) -> (37.0962, 62.0954)
  line L105 (34.2865, 63.1114) -> (34.2865, 62.0954)
  line L106 (37.0962, 63.1114) -> (34.2865, 63.1114)
  line L107 (37.0962, 62.0954) -> (37.0962, 63.1114)
  line L108 (31.7966, 44.45) -> (43.5019, 51.0525)
  line L109 (42.4624, 51.6596) -> (31.8107, 45.6515)
  line L110 (42.0481, 52.1761) -> (31.9218, 46.3281)
  line L111 (31.9218, 49.1234) -> (37.7054, 52.5185)
  line L112 (31.9218, 48.7095) -> (38.0845, 52.3272)
  line L113 (31.9218, 49.1234) -> (31.9218, 51.0535)
  line L114 (29.0948, 67.2715) -> (29.0948, 67.5351)
  line L115 (29.4758, 67.2715) -> (31.6066, 68.502)
  line L116 (29.0948, 67.5351) -> (31.6066, 68.9857)
  line L117 (31.6066, 65.8741) -> (31.6066, 68.502)
  line L118 (31.6066, 68.9857) -> (31.6066, 70.2564)
  circle A14 centre (29.2853, 63.9396) radius 0.3175
  arc A15 (29.0948, 64.6116) -> (29.4758, 64.6116) centre (29.2853, 63.9396) ccw
  line L119 (29.0948, 64.9028) -> (29.0948, 64.6116)
  line L120 (29.0948, 64.9028) -> (25.8093, 64.9028)
  line L121 (22.9961, 65.2838) -> (29.0948, 65.2838)
  line L122 (29.4758, 64.6116) -> (29.4758, 67.2715)
  line L123 (29.0948, 67.2715) -> (29.0948, 65.2838)
  line L124 (22.9961, 65.2838) -> (31.6066, 70.2564)
  line L125 (31.9876, 66.1004) -> (31.9876, 65.8741)
  line L126 (31.9911, 70.2625) -> (31.9911, 66.4814)
  line L127 (20.9808, 64.9373) -> (31.7409, 71.0066)
  circle A16 centre (31.7971, 65.0383) radius 0.4127
  line L128 (31.75, 72.2052) -> (19.9413, 65.5444)
  line L129 (20.9808, 52.1009) -> (20.9808, 64.9373)
  line L130 (19.9413, 65.5444) -> (19.9413, 51.51)
  circle A17 centre (31.7313, 51.824) radius 0.4127
  line L131 (31.5408, 46.3613) -> (21.4951, 52.278)
  line L132 (19.9413, 51.51) -> (31.7966, 44.45)
  line L133 (31.8107, 45.6515) -> (20.9808, 52.1009)
  line L134 (31.5408, 49.8815) -> (26.3439, 52.8489)
  line L135 (26.3439, 52.4415) -> (31.5408, 49.4741)
  line L136 (31.5408, 51.0535) -> (31.5408, 49.8815)
  arc A18 (31.9218, 51.0535) -> (31.5408, 51.0535) centre (31.7313, 51.824) ccw
  circle A19 centre (41.0606, 62.1232) radius 0.381
  line L137 (40.8701, 59.3346) -> (39.5527, 59.3346)
  line L138 (39.4243, 58.9536) -> (40.8701, 58.9536)
  line L139 (37.7054, 52.5185) -> (37.7054, 53.0908)
  circle A20 centre (37.8959, 53.9267) radius 0.4763
  line L140 (38.7282, 53.737) -> (42.0481, 53.737)
  line L141 (38.0845, 53.0941) -> (38.0845, 52.3272)
  arc A21 (38.7317, 54.1172) -> (37.7054, 53.0908) centre (37.8959, 53.9267) ccw
  arc A22 (38.0845, 53.0941) -> (38.7282, 53.737) centre (37.8959, 53.9267) ccw
  line L142 (42.0481, 53.737) -> (42.0481, 52.1761)
  line L143 (43.5019, 51.0525) -> (43.5019, 65.3384)
  line L144 (42.4624, 64.7418) -> (42.4624, 51.6596)
  line L145 (41.2511, 61.3863) -> (41.2511, 54.1172)
  line L146 (39.4243, 58.9536) -> (38.6183, 59.7969)
  line L147 (39.5527, 59.3346) -> (38.9824, 59.9313)
  arc A23 (41.2511, 61.3863) -> (40.8701, 61.3863) centre (41.0606, 62.1232) ccw
  line L148 (38.3095, 61.5459) -> (38.3095, 62.5274)
  arc A24 (38.9824, 59.9313) -> (38.6905, 61.5459) centre (38.5, 60.6778) ccw
  line L149 (40.8701, 59.3346) -> (40.8701, 61.3863)
  line L150 (42.0481, 64.4224) -> (42.0481, 54.1172)
  line L151 (42.0481, 54.1172) -> (41.2511, 54.1172)
  line L152 (40.8701, 54.1172) -> (40.8701, 58.9536)
  line L153 (40.8701, 54.1172) -> (38.7317, 54.1172)
  arc A25 (38.3095, 61.5459) -> (38.6183, 59.7969) centre (38.5, 60.6778) ccw
  line L154 (43.5019, 65.3384) -> (31.75, 72.2052)
  line L155 (31.7409, 71.0066) -> (42.4624, 64.7418)
  line L156 (38.5023, 66.4814) -> (31.9911, 66.4814)
  line L157 (31.9876, 70.2646) -> (38.5023, 66.4814)
  line L158 (31.9911, 66.4814) -> (31.9911, 70.2625)
  line L159 (31.9911, 70.2625) -> (38.5023, 66.4814)
  line L160 (31.9911, 66.4814) -> (38.5023, 66.4814)
  line L161 (28.0615, 58.9484) -> (28.0615, 61.2883)
  line L162 (29.8151, 63.1194) -> (30.9581, 63.1194)
  line L163 (30.9581, 63.1194) -> (30.9581, 58.9484)
  line L164 (29.8151, 58.9484) -> (28.0615, 61.2883)
  line L165 (33.8556, 61.9764) -> (32.6087, 61.9764)
  line L166 (31.4657, 63.1194) -> (33.8556, 63.1194)
  line L167 (33.8556, 63.1194) -> (33.8556, 61.9764)
  line L168 (31.4657, 58.9484) -> (31.4657, 63.1194)
  line L169 (31.4657, 63.1194) -> (32.6087, 63.1194)
  line L170 (29.8151, 60.7795) -> (29.8151, 63.1194)
  line L171 (28.0615, 63.1194) -> (29.8151, 60.7795)
  line L172 (31.4657, 61.9764) -> (31.4657, 63.1194)
  line L173 (22.6601, 31.2964) -> (22.6651, 29.8066)
  line L174 (22.6665, 29.4256) -> (22.6651, 29.8066)
  line L175 (22.6507, 34.0285) -> (22.6587, 31.6774)
  line L176 (21.5243, 35.8431) -> (25.9921, 35.8584)
  line L177 (25.9908, 36.2394) -> (21.523, 36.2241)
  line L178 (22.2842, 29.8053) -> (21.5449, 29.8027)
  line L179 (21.5462, 29.4217) -> (22.2855, 29.4243)
  circle A26 centre (22.4578, 34.7329) radius 0.3493
  arc A27 (22.6507, 34.0285) -> (22.2697, 34.0272) centre (22.4578, 34.7329) ccw
  line L180 (22.2842, 29.8053) -> (22.2697, 34.0272)
  line L181 (21.523, 36.2241) -> (21.5243, 35.8431)
  line L182 (21.0767, 36.7309) -> (21.12, 24.0813)
  line L183 (19.9676, 23.5047) -> (19.9586, 37.4674)
  line L184 (21.5221, 36.4783) -> (21.5449, 29.8027)
  line L185 (26.9619, 31.6921) -> (22.6587, 31.6774)
  line L186 (22.6601, 31.2964) -> (26.9632, 31.3111)
  line L187 (26.9632, 31.3111) -> (26.9619, 31.6921)
  arc A28 (25.8644, 28.2691) -> (25.4834, 28.2678) centre (25.6715, 28.9736) ccw
  circle A29 centre (25.6715, 28.9736) radius 0.3493
  line L188 (31.8713, 16.6404) -> (19.9676, 23.5047)
  line L189 (21.12, 24.0813) -> (31.8964, 17.907)
  line L190 (23.0676, 23.4777) -> (31.6951, 18.5346)
  line L191 (29.165, 23.8796) -> (29.164, 24.1708)
  line L192 (29.1731, 21.5109) -> (29.1663, 23.4986)
  line L193 (29.1731, 21.5109) -> (29.174, 21.2473)
  line L194 (29.545, 24.1721) -> (29.5541, 21.5122)
  line L195 (29.5541, 21.5122) -> (31.6891, 20.289)
  line L196 (29.174, 21.2473) -> (31.6907, 19.8053)
  line L197 (31.6801, 22.9169) -> (31.6891, 20.289)
  line L198 (31.6907, 19.8053) -> (31.6951, 18.5346)
  line L199 (32.0796, 18.5298) -> (32.0667, 22.3109)
  line L200 (32.0618, 22.6919) -> (32.0611, 22.9182)
  circle A30 centre (31.8677, 23.7534) radius 0.4127
  arc A31 (32.0611, 22.9182) -> (31.6801, 22.9169) centre (31.8677, 23.7534) ccw
  circle A32 centre (41.1212, 26.7001) radius 0.381
  arc A33 (40.9282, 27.4363) -> (41.3092, 27.4376) centre (41.1212, 26.7001) ccw
  line L201 (40.9212, 29.488) -> (40.9282, 27.4363)
  circle A34 centre (38.5556, 28.1368) radius 0.508
  line L202 (40.9212, 29.488) -> (39.6037, 29.4835)
  arc A35 (38.7491, 27.2693) -> (39.0355, 28.8849) centre (38.5556, 28.1368) ccw
  line L203 (39.6037, 29.4835) -> (39.0355, 28.8849)
  line L204 (39.474, 29.8641) -> (40.9199, 29.869)
  line L205 (39.474, 29.8641) -> (38.6709, 29.0181)
  line L206 (42.1166, 24.4043) -> (42.0813, 34.7095)
  line L207 (42.562, 24.1393) -> (42.5183, 36.9086)
  line L208 (43.6866, 37.5937) -> (43.6957, 23.5059)
  line L209 (41.3092, 27.4376) -> (41.2843, 34.7068)
  line L210 (40.9033, 34.7055) -> (40.9199, 29.869)
  line L211 (38.7601, 35.0783) -> (42.08, 35.0897)
  line L212 (40.9033, 34.7055) -> (38.7649, 34.6981)
  line L213 (26.9772, 27.2181) -> (25.868, 27.2143)
  line L214 (25.8693, 26.8333) -> (26.9785, 26.8371)
  line L215 (25.868, 27.2143) -> (25.8644, 28.2691)
  line L216 (25.868, 27.2143) -> (25.8682, 27.1538)
  line L217 (22.6739, 27.2564) -> (22.6665, 29.4256)
  line L218 (22.2855, 29.4243) -> (22.2934, 27.1057)
  line L219 (25.4834, 28.2678) -> (25.4952, 24.8108)
  line L220 (22.6739, 27.2564) -> (25.4952, 24.8108)
  line L221 (21.5462, 29.4217) -> (21.5636, 24.3395)
  line L222 (25.8795, 23.8684) -> (25.8693, 26.8333)
  line L223 (25.4985, 23.8671) -> (22.4066, 23.8565)
  line L224 (21.5636, 24.3395) -> (22.4066, 23.8565)
  line L225 (22.2934, 27.1057) -> (25.4969, 24.3288)
  line L226 (25.9921, 35.8584) -> (26.0007, 33.3235)
  line L227 (26.3804, 33.7058) -> (26.3728, 35.924)
  line L228 (25.9885, 36.9013) -> (25.9908, 36.2394)
  line L229 (26.3714, 36.3314) -> (26.3695, 36.9026)
  line L230 (26.9563, 33.3268) -> (26.955, 33.7078)
  line L231 (26.955, 33.7078) -> (26.3804, 33.7058)
  line L232 (25.9994, 33.7045) -> (26.0007, 33.3235)
  line L233 (26.0007, 33.3235) -> (26.3817, 33.3248)
  line L234 (26.0007, 33.3235) -> (26.9563, 33.3268)
  line L235 (26.954, 34.0219) -> (26.9505, 35.0379)
  line L236 (25.4819, 28.6948) -> (25.482, 28.6802)
  line L237 (25.4969, 24.3288) -> (25.4985, 23.8671)
  line L238 (30.5693, 35.0503) -> (30.8814, 34.2954)
  line L239 (29.2143, 34.0297) -> (28.097, 34.0258)
  line L240 (29.4263, 35.0464) -> (30.5693, 35.0503)
  line L241 (29.4263, 35.0464) -> (30.8931, 30.8743)
  line L242 (26.9505, 35.0379) -> (26.9648, 30.8608)
  line L243 (29.2108, 35.0457) -> (29.2143, 34.0297)
  line L244 (28.1078, 30.8647) -> (28.097, 34.0258)
  circle A36 centre (31.7568, 36.9673) radius 0.4127
  line L245 (31.9366, 40.0825) -> (38.1116, 36.4859)
  line L246 (31.938, 39.6686) -> (37.7332, 36.2932)
  line L247 (30.8814, 34.2954) -> (32.1514, 34.2998)
  line L248 (32.4805, 35.0569) -> (32.1514, 34.2998)
  line L249 (33.9429, 35.0619) -> (35.9079, 35.0686)
  line L250 (31.081, 33.4233) -> (31.9594, 33.4263)
  line L251 (31.523, 32.3682) -> (31.081, 33.4233)
  line L252 (31.9594, 33.4263) -> (31.523, 32.3682)
  line L253 (35.0384, 34.1097) -> (35.6249, 34.1117)
  line L254 (35.041, 33.3599) -> (35.6356, 33.3619)
  circle A37 centre (37.9285, 34.8858) radius 0.4763
  arc A38 (37.7351, 35.7209) -> (38.7649, 34.6981) centre (37.9285, 34.8858) ccw
  arc A39 (36.3784, 32.8027) -> (35.9079, 35.0686) centre (35.9728, 33.9003) ccw
  line L255 (33.9054, 29.8503) -> (33.9093, 28.7073)
  line L256 (31.938, 39.6686) -> (31.9446, 37.7385)
  line L257 (35.0461, 31.8563) -> (35.4817, 31.8578)
  line L258 (32.4805, 35.0569) -> (33.6235, 35.0608)
  line L259 (35.0438, 32.5368) -> (35.4794, 32.5383)
  line L260 (35.0384, 34.1097) -> (35.041, 33.3599)
  arc A40 (35.6356, 33.3619) -> (35.6249, 34.1117) centre (35.597, 33.7363) ccw
  line L261 (35.0438, 32.5368) -> (35.0461, 31.8563)
  arc A41 (35.4817, 31.8578) -> (35.4794, 32.5383) centre (35.375, 32.1977) ccw
  arc A42 (35.9222, 30.8915) -> (36.3784, 32.8027) centre (35.6902, 31.9569) ccw
  line L262 (33.9572, 30.8847) -> (35.9222, 30.8915)
  line L263 (33.6235, 35.0608) -> (32.1631, 30.8786)
  line L264 (33.9429, 35.0619) -> (33.9572, 30.8847)
  line L265 (42.0813, 34.7095) -> (41.2843, 34.7068)
  line L266 (42.08, 35.0897) -> (42.0747, 36.6505)
  line L267 (26.9648, 30.8608) -> (28.1078, 30.8647)
  line L268 (28.1256, 25.6594) -> (26.9826, 25.6555)
  line L269 (26.9785, 26.8371) -> (26.9772, 27.2181)
  line L270 (26.9826, 25.6555) -> (26.9683, 29.8265)
  line L271 (26.9683, 29.8265) -> (28.1113, 29.8304)
  line L272 (28.1113, 29.8304) -> (28.1193, 27.4905)
  line L273 (28.1256, 25.6594) -> (29.8712, 28.0053)
  line L274 (29.8649, 29.8364) -> (28.1193, 27.4905)
  line L275 (29.8712, 28.0053) -> (29.8792, 25.6654)
  line L276 (31.0079, 29.8403) -> (29.8649, 29.8364)
  line L277 (31.0222, 25.6693) -> (31.0079, 29.8403)
  circle A43 centre (29.3522, 24.8434) radius 0.3175
  line L278 (29.8792, 25.6654) -> (31.0222, 25.6693)
  arc A44 (29.545, 24.1721) -> (29.164, 24.1708) centre (29.3522, 24.8434) ccw
  line L279 (38.3728, 25.9055) -> (38.3837, 22.7135)
  line L280 (38.7647, 22.7148) -> (38.7491, 27.2693)
  line L281 (38.3681, 27.268) -> (38.3715, 26.2865)
  circle A45 centre (26.1761, 37.735) radius 0.4762
  arc A46 (26.3695, 36.9026) -> (25.9885, 36.9013) centre (26.1761, 37.735) ccw
  line L282 (28.0935, 35.0418) -> (26.9505, 35.0379)